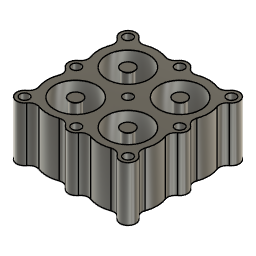
Cast_H+Lid (Autodesk Fusion 360 design; units mm, degrees)
Autodesk Fusion 360 part; units mm, degrees
note: some values were not read from the file. Chosen so that the rebuilt part matches the saved one: which bodies a step acts on.
sketch "Esboço1" plane through (0, 0, 0) normal (0, 0, 1) x (1, 0, 0) in component "Cast_Bottom"
  arc A0 (21.549, 0) -> (18.049, 0) centre (19.799, 0) ccw
  arc A1 (0, -18.049) -> (0, -21.549) centre (0, -19.799) ccw
  arc A2 (20.3179, 6.0337) -> (20.3179, 13.7653) centre (9.8995, 9.8995) ccw
  arc A3 (-18.049, 0) -> (-21.549, 0) centre (-19.799, 0) ccw
  circle A4 centre (19.799, 19.799) radius 1.75
  circle A5 centre (-19.799, -19.799) radius 1.75
  circle A6 centre (-19.799, 19.799) radius 1.75
  arc A7 (0, 21.549) -> (0, 18.049) centre (0, 19.799) ccw
  circle A8 centre (0, 0) radius 1.75
  arc A9 (-21.549, 0) -> (-18.049, 0) centre (-19.799, 0) ccw
  arc A10 (2.495, 21.4648) -> (0, 22.799) centre (0, 19.799) ccw
  arc A11 (-21.4648, 2.495) -> (-20.3179, 6.0337) centre (-23.1305, 4.9901) ccw
  arc A12 (-13.7653, -20.3179) -> (-17.304, -21.4648) centre (-14.8089, -23.1305) ccw
  arc A13 (13.7653, 20.3179) -> (17.304, 21.4648) centre (14.8089, 23.1305) ccw
  arc A14 (21.4648, 17.304) -> (20.3179, 13.7653) centre (23.1305, 14.8089) ccw
  arc A15 (-2.495, -21.4648) -> (-6.0337, -20.3179) centre (-4.9901, -23.1305) ccw
  arc A16 (13.7653, 20.3179) -> (6.0337, 20.3179) centre (9.8995, 9.8995) ccw
  arc A17 (20.3179, 6.0337) -> (21.4648, 2.495) centre (23.1305, 4.9901) ccw
  arc A18 (6.0337, -20.3179) -> (13.7653, -20.3179) centre (9.8995, -9.8995) ccw
  arc A19 (-21.4648, 2.495) -> (-22.799, 0) centre (-19.799, 0) ccw
  arc A20 (22.799, 0) -> (21.4648, 2.495) centre (19.799, 0) ccw
  arc A21 (17.304, -21.4648) -> (21.4648, -17.304) centre (19.799, -19.799) ccw
  arc A22 (0, 18.049) -> (0, 21.549) centre (0, 19.799) ccw
  arc A23 (-20.3179, 13.7653) -> (-20.3179, 6.0337) centre (-9.8995, 9.8995) ccw
  arc A24 (18.049, 0) -> (21.549, 0) centre (19.799, 0) ccw
  circle A25 centre (19.799, -19.799) radius 1.75
  arc A26 (0, -21.549) -> (0, -18.049) centre (0, -19.799) ccw
  arc A27 (20.3179, -13.7653) -> (20.3179, -6.0337) centre (9.8995, -9.8995) ccw
  arc A28 (0, -22.799) -> (2.495, -21.4648) centre (0, -19.799) ccw
  arc A29 (20.3179, -13.7653) -> (21.4648, -17.304) centre (23.1305, -14.8089) ccw
  arc A30 (21.4648, -2.495) -> (22.799, 0) centre (19.799, 0) ccw
  arc A31 (-22.799, 0) -> (-21.4648, -2.495) centre (-19.799, 0) ccw
  arc A32 (-17.304, 21.4648) -> (-21.4648, 17.304) centre (-19.799, 19.799) ccw
  arc A33 (6.0337, -20.3179) -> (2.495, -21.4648) centre (4.9901, -23.1305) ccw
  arc A34 (21.4648, -2.495) -> (20.3179, -6.0337) centre (23.1305, -4.9901) ccw
  arc A35 (-20.3179, -6.0337) -> (-20.3179, -13.7653) centre (-9.8995, -9.8995) ccw
  arc A36 (-20.3179, -6.0337) -> (-21.4648, -2.495) centre (-23.1305, -4.9901) ccw
  arc A37 (0, 22.799) -> (-2.495, 21.4648) centre (0, 19.799) ccw
  arc A38 (-21.4648, -17.304) -> (-17.304, -21.4648) centre (-19.799, -19.799) ccw
  arc A39 (-2.495, -21.4648) -> (0, -22.799) centre (0, -19.799) ccw
  arc A40 (-20.3179, 13.7653) -> (-21.4648, 17.304) centre (-23.1305, 14.8089) ccw
  arc A41 (-21.4648, -17.304) -> (-20.3179, -13.7653) centre (-23.1305, -14.8089) ccw
  arc A42 (-6.0337, 20.3179) -> (-13.7653, 20.3179) centre (-9.8995, 9.8995) ccw
  arc A43 (-13.7653, -20.3179) -> (-6.0337, -20.3179) centre (-9.8995, -9.8995) ccw
  arc A44 (2.495, 21.4648) -> (6.0337, 20.3179) centre (4.9901, 23.1305) ccw
  arc A45 (21.4648, 17.304) -> (17.304, 21.4648) centre (19.799, 19.799) ccw
  arc A46 (-17.304, 21.4648) -> (-13.7653, 20.3179) centre (-14.8089, 23.1305) ccw
  arc A47 (-6.0337, 20.3179) -> (-2.495, 21.4648) centre (-4.9901, 23.1305) ccw
  arc A48 (17.304, -21.4648) -> (13.7653, -20.3179) centre (14.8089, -23.1305) ccw
  circle A49 centre (-10, -10) radius 2
  line L0 (1.75, 0) -> (22.5, 0)
  line L1 (0, 1.75) -> (0, 22.5)
  dimension "d54" = 4
  dimension "d55" = 10
  dimension "d56" = 10
  measures "d54" diameter of A49
  measures "d55" distance of A49.centre L0
  measures "d56" distance of A49.centre L1
sketch "Esboço2" plane through (0, 0, 0) normal (0, 0, 1) x (1, 0, 0) in component "Cast_Bottom"
  circle A0 centre (-10, 10) radius 10.75
  line L0 (20, 0) -> (2.5, 0)
  circle A1 centre (10, 10) radius 10.75
  circle A2 centre (10, -10) radius 10.75
  circle A3 centre (-10, -10) radius 10.75
  line L1 (20, -20) -> (-20, -20)
  line L2 (-20, -20) -> (-20, 20)
  line L3 (-20, 20) -> (20, 20)
  line L4 (20, 20) -> (20, -20)
  line L5 (20, -20) -> (-20, 20) construction
  line L6 (-20, -20) -> (20, 20) construction
  circle A4 centre (20, 20) radius 1.75
  circle A5 centre (-20, 20) radius 1.75
  circle A6 centre (20, -20) radius 1.75
  circle A7 centre (20, 0) radius 1.75
  circle A8 centre (0, 0) radius 1.75
  circle A9 centre (-20, -20) radius 1.75
  circle A10 centre (0, 20) radius 1.75
  circle A11 centre (0, -20) radius 1.75
  circle A12 centre (-20, 0) radius 1.75
  circle A13 centre (-20, 20) radius 3
  circle A14 centre (0, 20) radius 3
  circle A15 centre (20, 20) radius 3
  circle A16 centre (20, 0) radius 3
  circle A17 centre (20, -20) radius 3
  circle A18 centre (0, -20) radius 3
  circle A19 centre (-20, -20) radius 3
  circle A20 centre (-20, 0) radius 3
  circle A21 centre (-10, 10) radius 2
  circle A22 centre (10, 10) radius 2
  circle A23 centre (-10, -10) radius 2
  circle A24 centre (10, -10) radius 2
  dimension "d23" = 21.5
  dimension "d24" = 10
  dimension "d25" = 10
  dimension "d26" = 21.5
  dimension "d27" = 21.5
  dimension "d28" = 21.5
  dimension "d29" = 40
  dimension "d30" = 40
  dimension "d31" = 3.5
  dimension "d32" = 3.5
  dimension "d33" = 3.5
  dimension "d34" = 3.5
  dimension "d35" = 3.5
  dimension "d36" = 3.5
  dimension "d37" = 3.5
  dimension "d38" = 3.5
  dimension "d39" = 3.5
  dimension "d40" = 1.25
  dimension "d41" = 1.25
  dimension "d42" = 1.25
  dimension "d43" = 1.25
  dimension "d44" = 1.25
  dimension "d45" = 1.25
  dimension "d46" = 1.25
  dimension "d47" = 1.25
  dimension "d48" = 4
  dimension "d49" = 4
  dimension "d50" = 4
  dimension "d51" = 4
  constraint horizontal L1
  constraint perpendicular L1 L2
  constraint parallel L1 L3
  constraint parallel L2 L4
  constraint coincident L5 A8.centre
  constraint coincident L6 A8.centre
  constraint coincident A8.centre origin
  constraint coincident L2.end L3.start
  constraint coincident L3.end L4.start
  constraint coincident L1.start L4.end
  constraint coincident L1.end L2.start
  constraint midpoint L3 A10.centre
  constraint midpoint L4 L0.start
  constraint midpoint L2 A12.centre
  constraint midpoint L1 A11.centre
  constraint concentric A0 A21
  constraint concentric A1 A22
  constraint concentric A3 A23
  constraint concentric A2 A24
  measures "d23" diameter of A0
  measures "d24" horizontal distance of A8.centre A0.centre
  measures "d25" distance of A0.centre L0
  measures "d26" diameter of A1
  measures "d27" diameter of A3
  measures "d28" diameter of A2
  measures "d29" distance of L2.end L3.end
  measures "d30" distance of L1.end L2.end
  measures "d31" diameter of A4
  measures "d32" diameter of A5
  measures "d33" diameter of A6
  measures "d34" diameter of A7
  measures "d35" diameter of A8
  measures "d36" diameter of A9
  measures "d37" diameter of A10
  measures "d38" diameter of A11
  measures "d39" diameter of A12
  measures "d48" diameter of A21
  measures "d49" diameter of A22
  measures "d50" diameter of A23
  measures "d51" diameter of A24
sketch "Esboço1 (2)" plane through (0, 0, 0) normal (0, 0, 1) x (1, 0, 0) in component "Rubber_Rolls"
  circle A0 centre (0, 0) radius 2
  circle A1 centre (0, 0) radius 8.5
  line L0 (0, 2.5) -> (0, 20)
  dimension "d1" = 4
  dimension "d2" = 17
  constraint concentric A0 A1
  measures "d1" diameter of A0
  measures "d2" diameter of A1
sketch "Esboço4" plane through (0, 0, 0) normal (0, 1, 0) x (1, 0, 0) in component "Rubber_Rolls"
  line L0 (0, 0) -> (2, 0)
  line L1 (2, 0) -> (2, -19)
  line L2 (2, -19) -> (0, -19)
  line L3 (0, -19) -> (0, 0)
  line L4 (2, -19) -> (8.5, -19)
  line L5 (2, 0) -> (8.5, 0)
  circle A0 centre (-53.2738, -9.5) radius 62.5
  dimension "d14" = 19
  dimension "d15" = 6.5
  dimension "d16" = 6.5
  dimension "d17" = 125
  constraint horizontal L0
  constraint vertical L1
  constraint horizontal L2
  constraint vertical L3
  constraint coincident L0.start L3.end
  constraint perpendicular L1 L4
  constraint perpendicular L1 L5
  constraint coincident L4.end A0
  constraint coincident L5.end A0
  measures "d14" distance of L0.start L2.end
  measures "d15" distance of L1.end L4.end
  measures "d16" distance of L0.end L5.end
  measures "d17" diameter of A0
revolve "Revolucionar2" add sketch "Esboço4" angle 360 about axis through (0, 0, 19) along (0, 0, -1) contours L1 L4 L5 A0 makes body 1 in component "Rubber_Rolls"
fillet "Arredondamento1" radius 0.5 4 edges at (-1.8647, -0.7232, 19) (-1.8647, -0.7232, 0) (-7.9248, -3.0737, 19) (-7.9248, -3.0737, 0) on bodies 1 in component "Rubber_Rolls"
copy_body "Copiar e colar corpos4" bodies 1 makes body 2 in component "Rubber_Rolls"
move_body "Mover4" bodies 2 to x (1, 0, 0) y (0, 1, 0) z (0, 0, 1) at (20, 0, 0) in component "Rubber_Rolls"
copy_body "Copiar e colar corpos5" bodies 1 2 makes body 3 makes body 4 in component "Rubber_Rolls"
move_body "Mover5" bodies 3 4 to x (1, 0, 0) y (0, 1, 0) z (0, 0, 1) at (0, -20, 0) in component "Rubber_Rolls"
extrude "Extrusão1" add sketch "Esboço1" along normal up to surface (18.7904 mm away) separate body contours A2 A10 A11 A12 A13 A14 A15 A16 A17 A18 A19 A20 A21 A23 A27 A28 A29 A30 A31 A32 A33 A34 A35 A36 A37 A38 A39 A40 A41 A42 A43 A44 A45 A46 A47 A48 | A49 makes body 5 in component "Cast_Bottom"
combine "Combinar1" operation cut target body 5 tool bodies 1 2 3 4 body 1 seen with x (1, 0, 0) y (0, 1, 0) z (0, 0, 1) at (-9.7956, 9.7559, -0.2096) body 2 seen with x (1, 0, 0) y (0, 1, 0) z (0, 0, 1) at (-9.7956, 9.7559, -0.2096) body 3 seen with x (1, 0, 0) y (0, 1, 0) z (0, 0, 1) at (-9.7956, 9.7559, -0.2096) body 4 seen with x (1, 0, 0) y (0, 1, 0) z (0, 0, 1) at (-9.7956, 9.7559, -0.2096) keep tools makes body 6 at (-7.7981, 9.8556, 6.2904) makes body 7 at (-7.7981, -10.1444, 6.2904) makes body 8 at (12.2019, 9.8556, 6.2904) makes body 9 at (12.2019, -10.1444, 6.2904) in component "Cast_Bottom"
extrude "Extrusão2" add sketch "Esboço1" against normal blind 2 contours A2 A10 A11 A12 A13 A14 A15 A16 A17 A18 A19 A20 A21 A23 A27 A28 A29 A30 A31 A32 A33 A34 A35 A36 A37 A38 A39 A40 A41 A42 A43 A44 A45 A46 A47 A48 | A49 bodies 5 in component "Cast_Bottom"
component "Rubber_Rolls" placed x (1, 0, 0) y (0, 1, 0) z (0, 0, 1) at (-9.7956, 9.7559, -0.2096)
component "Cast_Bottom" placed x (1, 0, 0) y (0, 1, 0) z (0, 0, 1) at (0, 0, 0)
equation "d16 = d15"
equation "d26 = d23"
equation "d27 = d23"
equation "d28 = d23"
named bodies: "Roll_1", "Roll_2", "Roll_1 (1)", "Roll_1 (1) (1)", "Roll_3", "Roll_4"
